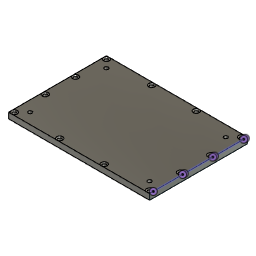
Base cover (Autodesk Fusion 360 design; units mm, degrees)
Autodesk Fusion 360 part; units mm, degrees
note: some values were not read from the file. Set by a fixed rule: which sketch regions a step uses.
sketch "Szkic1" plane through (0, 0, 0) normal (0, 0, 1) x (1, 0, 0)
  line L0 (0, 0) -> (196, 0)
  line L1 (196, 0) -> (196, 136)
  line L2 (196, 136) -> (0, 136)
  line L3 (0, 136) -> (0, 0)
  dimension "d1" = 196
  dimension "d2" = 136
  constraint horizontal L0
  constraint vertical L1
  constraint horizontal L2
  constraint vertical L3
  constraint coincident L0.start L3.end
  measures "d1" distance of L0.start L0.end
  measures "d2" distance of L0.start L2.end
extrude "Wyciągnięcie proste1" add sketch "Szkic1" along normal blind 8
sketch "Szkic2" plane through (0, 0, 8) normal (0, 0, 1) x (-1, 0, 0)
  line L0 (0, -136) -> (0, 0)
  line L1 (0, 0) -> (-196, 0)
  line L2 (-196, 0) -> (-196, -136)
  line L3 (-196, -136) -> (0, -136)
  line L4 (0, 0) -> (-4, 0)
  circle A0 centre (-4, -4) radius 2.65
  line L5 (-4, -4) -> (-4, -47)
  circle A1 centre (-4, -47) radius 2.65
  line L6 (-4, -47) -> (-4, -89)
  line L7 (-4, -89) -> (-4, -132)
  line L8 (-4, -132) -> (-67, -132)
  line L9 (-67, -132) -> (-129, -132)
  line L10 (-129, -132) -> (-192, -132)
  line L11 (-192, -132) -> (-192, -89)
  line L12 (-192, -89) -> (-192, -47)
  line L13 (-192, -47) -> (-192, -4)
  line L14 (-192, -4) -> (-129, -4)
  line L15 (-129, -4) -> (-67, -4)
  line L16 (-67, -4) -> (-4, -4)
  circle A2 centre (-4, -89) radius 2.65
  circle A3 centre (-4, -132) radius 2.65
  circle A4 centre (-67, -132) radius 2.65
  circle A5 centre (-129, -132) radius 2.65
  circle A6 centre (-192, -132) radius 2.65
  circle A7 centre (-192, -89) radius 2.65
  circle A8 centre (-192, -47) radius 2.65
  circle A9 centre (-192, -4) radius 2.65
  circle A10 centre (-129, -4) radius 2.65
  circle A11 centre (-67, -4) radius 2.65
  dimension "d5" = 5.3
  dimension "d6" = 43
  dimension "d7" = 5.3
  dimension "d8" = 42
  dimension "d9" = 43
  dimension "d10" = 63
  dimension "d11" = 62
  dimension "d12" = 63
  dimension "d13" = 43
  dimension "d14" = 42
  dimension "d15" = 43
  dimension "d16" = 63
  dimension "d17" = 62
  dimension "d18" = 5.3
  dimension "d19" = 5.3
  dimension "d20" = 5.3
  dimension "d21" = 5.3
  dimension "d22" = 5.3
  dimension "d23" = 5.3
  dimension "d24" = 5.3
  dimension "d25" = 5.3
  dimension "d26" = 5.3
  dimension "d27" = 5.3
  constraint coincident L0.end L1.start
  constraint coincident L1 L4.end
  constraint perpendicular L0 L4
  constraint coincident A0.centre L5.start
  constraint vertical L5
  constraint coincident L5.end A1.centre
  constraint parallel L5 L6
  constraint parallel L6 L7
  constraint perpendicular L7 L8
  constraint perpendicular L7 L9
  constraint perpendicular L7 L10
  constraint perpendicular L10 L11
  constraint perpendicular L10 L12
  constraint perpendicular L10 L13
  constraint perpendicular L11 L14
  constraint perpendicular L11 L15
  constraint coincident L6.end L7.start
  constraint coincident L7.end L8.start
  constraint coincident L8.end L9.start
  constraint coincident L9.end L10.start
  constraint coincident L10.end L11.start
  constraint coincident L11.end L12.start
  constraint coincident L12.end L13.start
  constraint coincident L13.end L14.start
  constraint coincident L14.end L15.start
  constraint coincident L15.end L16.start
  measures "d5" diameter of A0
  measures "d6" distance of A0.centre L5.end
  measures "d7" diameter of A1
  measures "d8" distance of L5.end L6.end
  measures "d9" distance of L6.end L7.end
  measures "d10" distance of L7.end L8.end
  measures "d11" distance of L8.end L9.end
  measures "d12" distance of L9.end L10.end
  measures "d13" distance of L10.end L11.end
  measures "d14" distance of L11.end L12.end
  measures "d15" distance of L12.end L13.end
  measures "d16" distance of L13.end L14.end
  measures "d17" distance of L14.end L15.end
  measures "d18" diameter of A2
  measures "d19" diameter of A3
  measures "d20" diameter of A4
  measures "d21" diameter of A5
  measures "d22" diameter of A6
  measures "d23" diameter of A7
  measures "d24" diameter of A8
  measures "d25" diameter of A9
  measures "d26" diameter of A10
  measures "d27" diameter of A11
extrude "Wyciągnięcie proste2" cut sketch "Szkic2" against normal blind 8 contours A0 L5 L16 | A0 L5 L16 | L15 L16 A11 | L15 L16 A11 | L5 A1 L6 | L5 A1 L6 | L14 L15 A10 | L14 L15 A10 | L6 L7 A2 | L6 L7 A2 | L13 L14 A9 | L13 L14 A9 | L7 L8 A3 | L7 L8 A3 | L12 L13 A8 | L12 L13 A8 | L8 L9 A4 | L8 L9 A4 | L11 L12 A7 | L11 L12 A7 | L9 L10 A5 | L9 L10 A5 | L10 L11 A6 | L10 L11 A6
chamfer "Fazowanie1" distance 1.5 angle 45 12 edges at (6.4707, 131.0417, 8) (6.4707, 88.0417, 8) (6.4707, 46.0417, 8) (6.4707, 3.0417, 8) (69.4707, 3.0417, 8) (69.4707, 131.0417, 8) (131.4707, 131.0417, 8) (194.4707, 131.0417, 8) (194.4707, 88.0417, 8) (194.4707, 46.0417, 8) (194.4707, 3.0417, 8) (131.4707, 3.0417, 8)
sketch "Szkic3" plane through (196, 0, 0) normal (1, 0, 0) x (0, 1, 0)
  line L0 (2.8943, 8) -> (0, 8)
  line L1 (0, 8) -> (0, 0)
  line L2 (0, 0) -> (136, 0)
  line L3 (136, 0) -> (136, 8)
  spline S0 degree 2 poles (2.8943, 8) (4, 7.7054) (5.1057, 8) knots 0 0 0 0.223159 0.223159 0.223159 weights 1 1.0375 1
  line L4 (136, 8) -> (133.1057, 8)
  spline S1 degree 2 poles (130.8943, 8) (132, 7.7054) (133.1057, 8) knots 0 0 0 0.223159 0.223159 0.223159 weights 1 1.0375 1
  line L5 (130.8943, 8) -> (90.1057, 8)
  spline S2 degree 2 poles (87.8943, 8) (89, 7.7054) (90.1057, 8) knots 0 0 0 0.223159 0.223159 0.223159 weights 1 1.0375 1
  line L6 (87.8943, 8) -> (48.1057, 8)
  spline S3 degree 2 poles (45.8943, 8) (47, 7.7054) (48.1057, 8) knots 0 0 0 0.223159 0.223159 0.223159 weights 1 1.0375 1
  line L7 (45.8943, 8) -> (5.1057, 8)
sketch "Szkic4" plane through (0, 0, 0) normal (0, 0, -1) x (1, 0, 0)
  circle A0 centre (192, -89) radius 2.65
  circle A1 centre (4, -132) radius 2.65
  circle A2 centre (67, -4) radius 2.65
  circle A3 centre (4, -4) radius 2.65
  circle A4 centre (67, -132) radius 2.65
  circle A5 centre (192, -47) radius 2.65
  circle A6 centre (192, -132) radius 2.65
  circle A7 centre (4, -89) radius 2.65
  circle A8 centre (129, -4) radius 2.65
  circle A9 centre (4, -47) radius 2.65
  circle A10 centre (129, -132) radius 2.65
  circle A11 centre (192, -4) radius 2.65
  line L0 (0, 0) -> (0, -136)
  line L1 (0, -136) -> (196, -136)
  line L2 (196, -136) -> (196, 0)
  line L3 (196, 0) -> (0, 0)
  circle A12 centre (15.5, -60.5) radius 2.6
  circle A13 centre (181, -60.5) radius 2.6
  circle A14 centre (181, -98) radius 2.6
  circle A15 centre (15.5, -98) radius 2.6
  dimension "d35" = 5.2
  dimension "d36" = 5.2
  dimension "d37" = 5.2
  dimension "d38" = 5.2
  dimension "d42" = 37.5
  dimension "d43" = 165.5
  measures "d35" diameter of A12
  measures "d36" diameter of A13
  measures "d37" diameter of A14
  measures "d38" diameter of A15
  measures "d42" distance of A12.centre A15.centre
  measures "d43" distance of A12.centre A13.centre
extrude "Wyciągnięcie proste3" cut sketch "Szkic4" against normal blind 5.5 contours A12 | A13 | A14 | A15
sketch "Szkic5" plane through (0, 0, 8) normal (0, 0, 1) x (-1, 0, 0)
  line L0 (-130.1057, 0) -> (-190.8943, 0)
  line L1 (-196, -5.1057) -> (-196, -45.8943)
  line L2 (-190.8943, -136) -> (-130.1057, -136)
  line L3 (0, -130.8943) -> (0, -90.1057)
  circle A0 centre (-15, -15) radius 2.6
  circle A1 centre (-15, -121) radius 2.6
  circle A2 centre (-181, -121) radius 2.6
  circle A3 centre (-181, -15) radius 2.6
  arc A4 (-130.1057, 0) -> (-127.8943, 0) centre (-129, -4) ccw
  arc A5 (-196, -5.1057) -> (-190.8943, 0) centre (-192, -4) ccw
  arc A6 (-196, -48.1057) -> (-196, -45.8943) centre (-192, -47) ccw
  line L4 (-196, -48.1057) -> (-196, -87.8943)
  arc A7 (-196, -90.1057) -> (-196, -87.8943) centre (-192, -89) ccw
  line L5 (-196, -90.1057) -> (-196, -130.8943)
  arc A8 (-190.8943, -136) -> (-196, -130.8943) centre (-192, -132) ccw
  arc A9 (-127.8943, -136) -> (-130.1057, -136) centre (-129, -132) ccw
  line L6 (-127.8943, -136) -> (-68.1057, -136)
  arc A10 (-65.8943, -136) -> (-68.1057, -136) centre (-67, -132) ccw
  line L7 (-65.8943, -136) -> (-5.1057, -136)
  arc A11 (0, -130.8943) -> (-5.1057, -136) centre (-4, -132) ccw
  arc A12 (0, -87.8943) -> (0, -90.1057) centre (-4, -89) ccw
  line L8 (0, -87.8943) -> (0, -48.1057)
  arc A13 (0, -45.8943) -> (0, -48.1057) centre (-4, -47) ccw
  line L9 (0, -45.8943) -> (0, -5.1057)
  arc A14 (-5.1057, 0) -> (0, -5.1057) centre (-4, -4) ccw
  line L10 (-5.1057, 0) -> (-65.8943, 0)
  arc A15 (-68.1057, 0) -> (-65.8943, 0) centre (-67, -4) ccw
  line L11 (-68.1057, 0) -> (-127.8943, 0)
  dimension "d44" = 5.2
  dimension "d45" = 166
  dimension "d46" = 106
  dimension "d47" = 5.2
  dimension "d48" = 5.2
  dimension "d49" = 5.2
  measures "d44" diameter of A0
  measures "d45" distance of A0.centre A3.centre
  measures "d46" distance of A0.centre A1.centre
  measures "d47" diameter of A1
  measures "d48" diameter of A2
  measures "d49" diameter of A3
extrude "Wyciągnięcie proste4" cut sketch "Szkic5" against normal blind 5.5 contours A0 | A1 | A2 | A3
